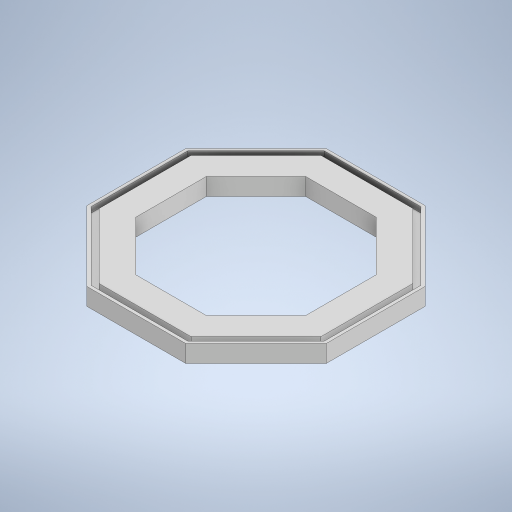
# Autodesk Inventor part: 팔각형 OV-PAM 5패턴 링 - 틈 너비 수정
Saved by Autodesk Inventor 2024 (Build 280153000, 153)
## iProperties
Created: 2023-06-19
Part Number: 팔각형 OV-PAM 5패턴 링 - 틈 너비 수정
Material: 일반
Document SubType Name: Modeling
Designer: jsw
Density: 1 g/cm^3
Appearance: 기본값
Author: jsw
Autodesk Inventor part; units mm, degrees
ref_plane "YZ Plane" through (0, 0, 0) normal (1, 0, 0) x (0, 1, 0)
ref_plane "XZ Plane" through (0, 0, 0) normal (0, 1, 0) x (-1, 0, 0)
ref_plane "XY Plane" through (0, 0, 0) normal (0, 0, 1) x (1, 0, 0)
sketch "스케치1" plane through (0, 0, 0) normal (0, 1, 0) x (-1, 0, 0)
  line L0 (-32.5919, 13.5) -> (-13.5, 32.5919)
  line L1 (-13.5, 32.5919) -> (13.5, 32.5919)
  line L2 (13.5, 32.5919) -> (32.5919, 13.5)
  line L3 (32.5919, 13.5) -> (32.5919, -13.5)
  line L4 (32.5919, -13.5) -> (13.5, -32.5919)
  line L5 (13.5, -32.5919) -> (-13.5, -32.5919)
  line L6 (-13.5, -32.5919) -> (-32.5919, -13.5)
  line L7 (-32.5919, -13.5) -> (-32.5919, 13.5)
  line L8 (34.5919, 14.3284) -> (34.5919, -14.3284)
  line L9 (34.5919, -14.3284) -> (14.3284, -34.5919)
  line L10 (14.3284, -34.5919) -> (-14.3284, -34.5919)
  line L11 (-14.3284, -34.5919) -> (-34.5919, -14.3284)
  line L12 (-34.5919, -14.3284) -> (-34.5919, 14.3284)
  line L13 (-34.5919, 14.3284) -> (-14.3284, 34.5919)
  line L14 (-14.3284, 34.5919) -> (14.3284, 34.5919)
  line L15 (14.3284, 34.5919) -> (34.5919, 14.3284)
  point P0 (0, 0)
  point P1 (0, 0)
  point P2 (0, 0)
  dimension "d0" = 27
  dimension "d1" = 2
  constraints: 32 end point, 2 coincident, 2 horizontal, 34 other
  measures "d0" distance of L2.end L3.end
  measures "d1" distance between parallel lines of L8 L3
extrude "돌출1" add sketch "스케치1" along normal blind 5 contours L0 L1 L2 L3 L4 L5 L6 L7 | L8 L9 L10 L11 L12 L13 L14 L15
sketch "스케치2" plane through (0, 5, 0) normal (0, 1, 0) x (1, 0, 0)
  line L0 (13.3, -32.109) -> (-13.3, -32.109)
  line L1 (-13.3, -32.109) -> (-32.109, -13.3)
  line L2 (-32.109, -13.3) -> (-32.109, 13.3)
  line L3 (-32.109, 13.3) -> (-13.3, 32.109)
  line L4 (-13.3, 32.109) -> (13.3, 32.109)
  line L5 (13.3, 32.109) -> (32.109, 13.3)
  line L6 (32.109, 13.3) -> (32.109, -13.3)
  line L7 (32.109, -13.3) -> (13.3, -32.109)
  line L8 (-13.9627, -33.709) -> (-33.709, -13.9627)
  line L9 (-33.709, -13.9627) -> (-33.709, 13.9627)
  line L10 (-33.709, 13.9627) -> (-13.9627, 33.709)
  line L11 (-13.9627, 33.709) -> (13.9627, 33.709)
  line L12 (13.9627, 33.709) -> (33.709, 13.9627)
  line L13 (33.709, 13.9627) -> (33.709, -13.9627)
  line L14 (33.709, -13.9627) -> (13.9627, -33.709)
  line L15 (13.9627, -33.709) -> (-13.9627, -33.709)
  point P0 (0, 0)
  point P1 (0, 0)
  point P2 (0, 0)
  dimension "d4" = 26.6
  dimension "d5" = 1.6
  constraints: 32 end point, 2 coincident, 2 horizontal, 34 other
  measures "d4" distance of L1.end L2.end
  measures "d5" distance between parallel lines of L2 L9
extrude "돌출2" cut sketch "스케치2" against normal blind 1.6
sketch "스케치3" plane through (0, 0, 0) normal (0, -1, 0) x (1, 0, 0)
  line L0 (-13.5, 32.5919) -> (13.5, 32.5919)
  line L1 (13.5, 32.5919) -> (32.5919, 13.5)
  line L2 (32.5919, 13.5) -> (32.5919, -13.5)
  line L3 (32.5919, -13.5) -> (13.5, -32.5919)
  line L4 (13.5, -32.5919) -> (-13.5, -32.5919)
  line L5 (-13.5, -32.5919) -> (-32.5919, -13.5)
  line L6 (-32.5919, -13.5) -> (-32.5919, 13.5)
  line L7 (-32.5919, 13.5) -> (-13.5, 32.5919)
  line L8 (-13.9971, 33.7919) -> (13.9971, 33.7919)
  line L9 (13.9971, 33.7919) -> (33.7919, 13.9971)
  line L10 (33.7919, 13.9971) -> (33.7919, -13.9971)
  line L11 (33.7919, -13.9971) -> (13.9971, -33.7919)
  line L12 (13.9971, -33.7919) -> (-13.9971, -33.7919)
  line L13 (-13.9971, -33.7919) -> (-33.7919, -13.9971)
  line L14 (-33.7919, -13.9971) -> (-33.7919, 13.9971)
  line L15 (-33.7919, 13.9971) -> (-13.9971, 33.7919)
  point P0 (0, 0)
  point P1 (0, 0)
  point P2 (0, 0)
  dimension "d8" = 27
  dimension "d9" = 1.2
  constraints: 32 end point, 2 coincident, 2 horizontal, 34 other
  measures "d8" distance of L0.start L0.end
  measures "d9" distance between parallel lines of L8 L0
extrude "돌출3" cut sketch "스케치3" against normal blind 1.6
sketch "스케치4" plane through (0, 5, 0) normal (0, 1, 0) x (1, 0, 0)
  line L0 (10.1934, -24.609) -> (-10.1934, -24.609)
  line L1 (-10.1934, -24.609) -> (-24.609, -10.1934)
  line L2 (-24.609, -10.1934) -> (-24.609, 10.1934)
  line L3 (-24.609, 10.1934) -> (-10.1934, 24.609)
  line L4 (-10.1934, 24.609) -> (10.1934, 24.609)
  line L5 (10.1934, 24.609) -> (24.609, 10.1934)
  line L6 (24.609, 10.1934) -> (24.609, -10.1934)
  line L7 (24.609, -10.1934) -> (10.1934, -24.609)
  line L8 (-32.109, 13.3) -> (-32.109, -13.3) projected
  point P0 (0, 0)
  point P1 (0, 0)
  dimension "d13" = 7.5
  constraints: 16 end point, 1 coincident, 1 horizontal, 17 other
  measures "d13" distance between parallel lines of L2 L8
extrude "돌출4" cut sketch "스케치4" against normal blind 5
